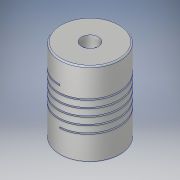
# Autodesk Inventor part: Shaft Coupler
Saved by Autodesk Inventor 2020.2 (Build 242310000, 310)
## iProperties
Created: 2018-09-02
Part Number: Shaft Coupler
Material: Aluminum 6061
Document SubType Name: Modeling
Designer: Richard
Density: 2.7 g/cm^3
Appearance: Aluminum - Flat
Author: Richard
Autodesk Inventor part; units mm, degrees
ref_plane "YZ Plane" through (0, 0, 0) normal (1, 0, 0) x (0, 1, 0)
ref_plane "XZ Plane" through (0, 0, 0) normal (0, 1, 0) x (-1, 0, 0)
ref_plane "XY Plane" through (0, 0, 0) normal (0, 0, 1) x (1, 0, 0)
sketch "Sketch1" plane through (0, 0, 0) normal (0, 1, 0) x (-1, 0, 0)
  circle A0 centre (0, 0) radius 9
  circle A1 centre (0, 0) radius 2.5
  dimension "d0" = 18
  dimension "d3" = 5
  constraints: 2 centre point, 2 coincident
  measures "d0" diameter of A0
  measures "d3" diameter of A1
extrude "Extrusion1" add sketch "Sketch1" along normal mid plane 25
sketch "Sketch2" plane through (0, 0, 0) normal (1, 0, 0) x (0, 1, 0)
  line L0 (6, 9) -> (5.6, 9)
  line L1 (5.6, 9) -> (5.6, 2.5)
  line L2 (5.6, 2.5) -> (6, 2.5)
  line L3 (6, 2.5) -> (6, 9)
  line L4 (-12.5, 9) -> (12.5, 9) projected
  line L5 (-12.5, 2.5) -> (12.5, 2.5) projected
  point P0 (0, 0)
  dimension "d4" = 0.4
  dimension "d5" = 6.5
  dimension "d6" = 6.5
  constraints: 8 end point, 2 collinear, 2 parallel, 1 horizontal, 1 perpendicular
  measures "d4" distance of L1.end L2.end
  measures "d5" distance of L2.end L0.start
  measures "d6" distance from line of L3 L4.end
coil "Coil1" sketch "Sketch2" operation cut axis through (0, -10, 0) along (0, -1, 0) pitch 2.2 turns 5 hand right
sketch "Sketch4" plane through (0, 0, 0) normal (1, 0, 0) x (0, 1, 0)
  line L0 (12.5, -9) -> (12.5, 9) projected
  line L1 (-12.5, 9) -> (-12.5, -9) projected
  point P0 (0, 0)
  point P1 (8.5, 0)
  point P2 (-8.5, 0)
  point P3 (12.5, 0)
  point P4 (-12.5, 0)
  dimension "d15" = 4
  dimension "d16" = 4
  constraints: 2 horizontal alignment, 2 midpoint
  measures "d15" distance from line of L0 point (8.5, 0)
  measures "d16" distance from line of L1 point (-8.5, 0)
hole "Hole1" at (0, 8.5, 0) at (0, -8.5, 0) direction (-1, 0, 0) diameter 2.459 end through all thread size "M3x0.5" class "6H" standard "ANSI Metric M Profile"
chamfer "Chamfer1" distance 0.381 angle 45 6 edges at (-8.9527, 7.6856, -0.9211) (-8.9529, 9.3156, -0.92) (-8.9156, 8.4999, 1.2295) (-8.9529, -7.6844, -0.92) (-8.9527, -9.3144, -0.9211) (-8.9156, -8.5001, 1.2295)
pattern_circular "Circular Pattern1" count 2 over 90 about axis through (0, 0, 0) along (0, -1, 0) of "Hole1", "Chamfer1"
fillet "Fillet1" radius 0.381 2 edges at (9, 12.5, 0) (9, -12.5, 0)
body "Solid1"
